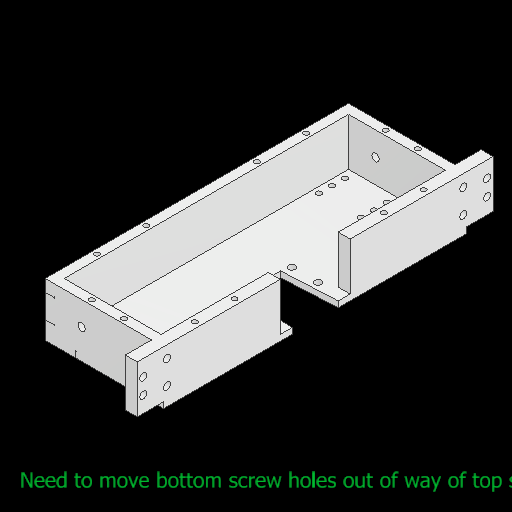
# Autodesk Inventor part: AfterComp1Chassis
Saved by Autodesk Inventor 2024.2 (Build 282272000, 272)
## iProperties
Created: 2021-02-15
Part Number: AfterComp1Chassis
Material: UHMW, White
Document SubType Name: Modeling
Designer: Esketitttttt
Density: 0.94 g/cm^3
Appearance: Smooth - White
Mass: 89.3613 g
Surface Area: 481.722 cm^2
Volume: 95.0653 cm^3
ThreadingScrew: 0.110 in
ThroughScrew: 0.150 in
Author: Esketitttttt
Autodesk Inventor part; units mm, degrees
ref_plane "YZ Plane" through (0, 0, 0) normal (1, 0, 0) x (0, 1, 0)
ref_plane "XZ Plane" through (0, 0, 0) normal (0, 1, 0) x (-1, 0, 0)
sketch "BasePlan" plane through (0, 0, 0) normal (0, 1, 0) x (-1, 0, 0)
  line L0 (0, 0) -> (-51.64, 0)
  line L1 (-51.64, 0) -> (-51.64, -24.585)
  line L2 (-51.64, -24.585) -> (0, -24.585)
  line L3 (0, -24.585) -> (0, 0)
  line L4 (0, 0) -> (-28.78, 0)
  line L5 (-28.78, 0) -> (-28.78, 63.5)
  line L6 (-28.78, 63.5) -> (0, 63.5)
  line L7 (0, 63.5) -> (0, 0)
  line L8 (-28.78, 63.5) -> (-51.64, 63.5)
  line L9 (-51.64, 63.5) -> (-51.64, 0)
  line L10 (-51.64, 0) -> (-28.78, 0)
  line L11 (-28.78, 0) -> (-28.78, 63.5)
  line L12 (0, 0) -> (0, -12.2925)
  line L13 (0, -12.2925) -> (8.9825, -12.2925) construction
  line L14 (-28.78, -24.585) -> (-28.78, -88.085)
  line L15 (-28.78, -88.085) -> (0, -88.085)
  line L16 (0, -88.085) -> (0, -24.585)
  line L17 (-28.78, -88.085) -> (-51.64, -88.085)
  line L18 (-51.64, -88.085) -> (-51.64, -24.585)
  line L19 (0, -88.085) -> (6.35, -88.085) construction
  line L20 (6.35, -88.085) -> (6.35, -94.435) construction
  line L21 (6.35, -94.435) -> (0, -94.435) construction
  line L22 (0, -94.435) -> (0, -88.085) construction
  line L23 (0, 63.5) -> (6.35, 63.5) construction
  line L24 (6.35, 63.5) -> (6.35, 69.85) construction
  line L25 (6.35, 69.85) -> (0, 69.85) construction
  line L26 (0, 69.85) -> (0, 63.5) construction
  line L27 (-51.64, -88.085) -> (-57.99, -88.085) construction
  line L28 (-57.99, -88.085) -> (-57.99, -94.435) construction
  line L29 (-57.99, -94.435) -> (-51.64, -94.435) construction
  line L30 (-51.64, -94.435) -> (-51.64, -88.085) construction
  line L31 (-51.64, 63.5) -> (-57.99, 63.5) construction
  line L32 (-57.99, 63.5) -> (-57.99, 69.85) construction
  line L33 (-57.99, 69.85) -> (-51.64, 69.85) construction
  line L34 (-51.64, 69.85) -> (-51.64, 63.5) construction
  line L35 (-57.99, 69.85) -> (-51.64, 69.85)
  line L36 (-51.64, 69.85) -> (-51.64, 0)
  line L37 (-51.64, 0) -> (-57.99, 0)
  line L38 (-57.99, 0) -> (-57.99, 69.85)
  line L39 (6.35, 69.85) -> (0, 69.85)
  line L40 (0, 69.85) -> (0, -94.435)
  line L41 (0, -94.435) -> (6.35, -94.435)
  line L42 (6.35, -94.435) -> (6.35, 69.85)
  line L43 (-51.64, 69.85) -> (0, 69.85)
  line L44 (0, 69.85) -> (0, 63.5)
  line L45 (0, 63.5) -> (-51.64, 63.5)
  line L46 (-51.64, 63.5) -> (-51.64, 69.85)
  line L47 (-51.64, -88.085) -> (0, -88.085)
  line L48 (0, -88.085) -> (0, -94.435)
  line L49 (0, -94.435) -> (-51.64, -94.435)
  line L50 (-51.64, -94.435) -> (-51.64, -88.085)
  line L51 (-57.99, -94.435) -> (-51.64, -94.435)
  line L52 (-51.64, -94.435) -> (-51.64, -24.585)
  line L53 (-51.64, -24.585) -> (-57.99, -24.585)
  line L54 (-57.99, -24.585) -> (-57.99, -94.435)
  line L55 (-51.64, -24.585) -> (-57.99, -24.585)
  line L56 (-57.99, -24.585) -> (-57.99, -30.935)
  line L57 (-57.99, -30.935) -> (-51.64, -30.935)
  line L58 (-51.64, -30.935) -> (-51.64, -24.585)
  line L59 (-51.64, 0) -> (-57.99, 0)
  line L60 (-57.99, 0) -> (-57.99, 6.35)
  line L61 (-57.99, 6.35) -> (-51.64, 6.35)
  line L62 (-51.64, 6.35) -> (-51.64, 0)
  line L63 (-51.64, 69.85) -> (-57.99, 69.85)
  line L64 (-57.99, 69.85) -> (-57.99, 82.55)
  line L65 (-57.99, 82.55) -> (-51.64, 82.55)
  line L66 (-51.64, 82.55) -> (-51.64, 69.85)
  line L67 (-57.99, -94.435) -> (-51.64, -94.435)
  line L68 (-57.99, -94.435) -> (-57.99, -107.135)
  line L69 (-57.99, -107.135) -> (-51.64, -107.135)
  line L70 (-51.64, -107.135) -> (-51.64, -94.435)
  line L71 (-51.64, -12.2925) -> (-28.78, -12.2925) construction
  line L72 (-28.78, -12.2925) -> (-28.78, -23.0875)
  line L73 (-28.78, -12.2925) -> (-28.78, -1.4975)
  line L74 (-57.99, 0) -> (-28.78, -1.4975)
  line L75 (-57.99, -24.585) -> (-28.78, -23.0875)
  line L76 (0, -94.435) -> (5.08, -94.435)
  line L77 (5.08, -94.435) -> (5.08, 69.85)
  line L78 (5.08, 69.85) -> (0, 69.85)
  line L79 (0, 69.85) -> (0, -94.435)
  line L80 (6.35, -88.085) -> (-51.64, -88.085)
  line L81 (-51.64, -88.085) -> (-51.64, -93.165)
  line L82 (-51.64, -93.165) -> (6.35, -93.165)
  line L83 (6.35, -93.165) -> (6.35, -88.085)
  line L84 (6.35, 63.5) -> (-51.64, 63.5)
  line L85 (-51.64, 63.5) -> (-51.64, 68.58)
  line L86 (-51.64, 68.58) -> (6.35, 68.58)
  line L87 (6.35, 68.58) -> (6.35, 63.5)
  line L88 (-57.99, -94.435) -> (-51.64, -94.435)
  line L89 (-51.64, -94.435) -> (-51.64, -93.165)
  line L90 (-51.64, -93.165) -> (-57.99, -93.165)
  line L91 (-57.99, -93.165) -> (-57.99, -94.435)
  line L92 (-51.64, 68.58) -> (-57.99, 68.58)
  line L93 (-57.99, 68.58) -> (-57.99, 69.85)
  line L94 (-57.99, 69.85) -> (-51.64, 69.85)
  line L95 (-51.64, 69.85) -> (-51.64, 68.58)
  point P0 (0, -88.085)
  point P1 (-51.64, 6.35)
  point P2 (-51.64, -30.935)
  point P3 (5.08, -93.165)
  point P4 (5.08, 68.58)
  dimension "d3" = 28.78
  dimension "d5" = 22.86
  dimension "d6" = 24.585
  dimension "d7" = 63.5
  dimension "d8" = 51.64
  dimension "d9" = 51.64
  dimension "d10" = 12.2925
  dimension "d12" = 6.35
  dimension "d88" = 6.35
  dimension "d89" = 6.35
  dimension "d90" = 6.35
  dimension "d158" = 164.285
  dimension "d210" = 12.7
  dimension "d219" = 22.86
  dimension "d220" = 10.795
  dimension "d255" = 6.35
  dimension "d256" = 5.08
  dimension "d261" = 5.08
  dimension "d262" = 5.08
  constraints: 192 end point, 40 parallel, 22 horizontal, 20 perpendicular, 10 symmetric about line, 8 point on line, 6 equal length, 2 midpoint, 2 vertical
  measures "d3" distance of L5.end L6.end
  measures "d5" distance of L5.end L8.end
  measures "d6" distance of L2.end L0.start
  measures "d7" distance of L6.end L0.start
  measures "d8" distance of L8.end L6.end
  measures "d9" distance of L1.end L2.end
  measures "d10" distance of L0.start L12.end
  measures "d12" distance of L19.end L20.end
  measures "d88" distance of L57.end L56.end
  measures "d89" distance of L56.end L55.end
  measures "d90" distance of L59.end L60.end
  measures "d158" distance of L41.end L24.end
  measures "d210" distance of L63.end L64.end
  measures "d219" distance of L71.start L71.end
  measures "d220" distance of L71.end L72.end
  measures "d255" distance between parallel lines of L40 L42
  measures "d256" distance of L78.end L77.end
  measures "d261" distance of L81.end L80.end
  measures "d262" distance of L84.end L85.end
extrude "BackWall" add sketch "BasePlan" along normal blind 25.4 contours L7 L84 L77 L80 L16 L3 | L40 L86 L77 L84 | L40 L39 L77 L86 | L84 L42 L80 L77 | L77 L86 L42 L84 | L80 L77 L82 L40 | L77 L39 L42 L86 | L80 L42 L82 L77 | L82 L77 L41 L40 | L82 L42 L41 L77
sketch "Sketch2" plane through (-6.35, 0, -94.435) normal (-1, 0, 0) x (0, 0, 1)
  line L0 (0, 0) -> (0, 25.4) construction
  line L1 (0, 0) -> (164.285, 0) construction
  line L2 (0, 0) -> (3.175, 0) construction
  line L3 (3.175, 0) -> (3.175, 6.35) construction
  line L4 (3.175, 6.35) -> (0, 6.35) construction
  line L5 (0, 6.35) -> (0, 0) construction
  line L6 (3.175, 0) -> (3.175, 19.05) construction
  line L7 (0, 25.4) -> (164.285, 25.4) projected
  line L8 (0, 25.4) -> (82.1425, 25.4) construction
  line L9 (82.1425, 25.4) -> (82.1425, 53.975) construction
  point P0 (94.435, 0)
  point P1 (6.35, 0)
  point P2 (161.11, 19.05)
  point P3 (161.11, 6.35)
  dimension "d25" = 6.35
  dimension "d26" = 25.4
  dimension "d27" = 3.175
  dimension "d28" = 6.35
  dimension "d29" = 19.05
  dimension "d30" = 164.285
  dimension "d31" = 82.1425
  constraints: 14 end point, 2 coincident, 2 parallel, 2 symmetric about line, 1 horizontal, 1 midpoint, 1 perpendicular, 1 point on line, 1 vertical
  measures "d25" distance of L0.start point (6.35, 0)
  measures "d26" distance of L0.start L0.end
  measures "d27" distance of L4.end L3.end
  measures "d28" distance of L3.end L2.end
  measures "d29" distance of L2.end L6.end
  measures "d30" distance of L0.end L7.end
  measures "d31" distance of L0.end L8.end
extrude "LeftSideWall" add sketch "BasePlan" along normal up to surface (25.4 mm away) contours L40 L82 L50 L17 L15 | L40 L49 L50 L82
extrude "RightSideWall" add sketch "BasePlan" along normal up to surface (25.4 mm away) contours L6 L8 L36 L86 L40 | L86 L36 L43 L40
hole "BackHoles" at (-6.35, 6.35, -91.26) at (-6.35, 19.05, -91.26) at (-6.35, 19.05, 66.675) at (-6.35, 6.35, 66.675) direction (1, 0, 0) diameter 3.81 depth 6.35
hole "Back Threading Holes" at (-6.35, 6.35, -91.26) at (-6.35, 19.05, -91.26) at (-6.35, 19.05, 66.675) at (-6.35, 6.35, 66.675) direction (1, 0, 0) diameter 2.794 depth 12.7 tip angle 118
extrude "RightFrontWall" add sketch "BasePlan" along normal up to surface (25.4 mm away) contours L61 L38 L92 L36 L9 | L92 L38 L35 L36 | L35 L64 L65 L66
extrude "LeftFrontWall" add sketch "BasePlan" along normal up to surface (25.4 mm away) contours L18 L50 L90 L54 L57 | L50 L51 L54 L90 | L70 L69 L68 L51
extrude "BottomUHMW" add sketch "BasePlan" against normal blind 3.175 contours L3 L2 L1 L75 L72 L73 L74 L0 | L7 L84 L77 L80 L16 L3 | L0 L5 L6 L7 | L0 L9 L8 L5 | L6 L8 L36 L86 L40 | L40 L86 L77 L84 | L37 L38 L61 L9 | L1 L74 L37 | L16 L15 L14 L2 | L86 L36 L43 L40 | L40 L39 L77 L86 | L84 L42 L80 L77 | L77 L86 L42 L84 | L61 L38 L92 L36 L9 | L14 L17 L18 L2 | L40 L82 L50 L17 L15 | L80 L77 L82 L40 | L92 L38 L35 L36 | L77 L39 L42 L86 | L80 L42 L82 L77 | L1 L53 L75 | L18 L57 L54 L53 | L82 L77 L41 L40 | L40 L49 L50 L82 | L82 L42 L41 L77 | L18 L50 L90 L54 L57 | L50 L51 L54 L90
sketch "Sketch4" plane through (0, 25.4, 0) normal (0, -1, 0) x (1, 0, 0)
  line L0 (-4.7625, -65.2173) -> (-4.7625, -63.6933) construction
  line L1 (-4.7625, -65.2173) -> (-4.7625, -63.6933) construction
  line L2 (0, -94.435) -> (0, -88.085) construction
  line L3 (-6.35, -96.4725) -> (-6.35, -94.435) construction
  line L4 (-6.35, -91.71) -> (-6.35, -96.4725) construction
  line L5 (0, 63.5) -> (0, -88.085)
  line L6 (0, -12.2925) -> (-7.0758, -12.2925)
  line L7 (54.815, -30.935) -> (57.99, -30.935) construction
  line L8 (57.99, -30.935) -> (57.99, -52.1017) construction
  line L9 (57.99, -52.1017) -> (54.815, -52.1017) construction
  line L10 (54.815, -52.1017) -> (54.815, -30.935) construction
  line L11 (54.815, -78.0308) -> (54.815, -73.2683) construction
  line L12 (-6.35, -94.435) -> (57.99, -94.435)
  line L13 (-6.35, -94.435) -> (57.99, -94.435) projected
  line L14 (-6.35, -94.435) -> (-3.1992, -94.435)
  line L15 (-2.54, -94.435) -> (-2.54, -68.1125) construction
  line L16 (51.64, -88.085) -> (0, -88.085) projected
  line L17 (-2.54, -94.435) -> (-2.54, -41.79) construction
  line L18 (57.99, -94.435) -> (57.99, -24.585) projected
  line L19 (57.99, -30.935) -> (51.64, -30.935) projected
  line L20 (-6.35, -94.435) -> (-6.35, 69.85) projected
  line L21 (-6.35, -94.435) -> (0, -94.435)
  point P0 (-2.54, 43.5275)
  point P1 (50.37, -94.435)
  point P2 (-2.54, 17.205)
  point P3 (57.99, 27.5167)
  point P4 (54.815, 48.6833)
  point P5 (57.99, -30.9122)
  point P6 (54.815, 27.5167)
  dimension "d104" = 4.7625
  dimension "d119" = 26.3225
  dimension "d121" = 82.1425
  dimension "d132" = 52.645
  dimension "d160" = 63.5
  dimension "d161" = 21.1667
  dimension "d162" = 21.1667
  dimension "d195" = 0
  dimension "d257" = 2.54
  dimension "d258" = 164.285
  constraints: 34 end point, 6 coincident, 5 point on line, 5 symmetric about line, 3 midpoint, 3 vertical, 2 parallel, 2 perpendicular, 1 collinear, 1 horizontal, 1 other
  measures "d104" distance of L11.start L11.end
  measures "d119" distance of L15.start L15.end
  measures "d121" distance between parallel lines of L12 L6
  measures "d132" distance of L15.start L17.end
  measures "d160" vertical distance of L7.end point (50.37, -94.435)
  measures "d161" vertical distance of point (54.815, -73.268) point (50.37, -94.435)
  measures "d162" distance of L7.end point (57.99, -52.102)
  measures "d195" distance between parallel lines of L10 L11
  measures "d257" distance between parallel lines of L5 L17
  measures "d258" distance of L3.end L20.end
hole "NewTopHoles" at (-2.54, 25.4, 43.5275) at (-2.54, 25.4, -68.1125) at (54.815, 25.4, -73.2683) at (-2.54, 25.4, -41.79) at (-2.54, 25.4, 17.205) at (54.815, 25.4, 48.6833) at (54.815, 25.4, -52.1017) at (54.815, 25.4, 27.5167) direction (0, -1, 0) diameter 2.794 depth 12.7 tip angle 118
sketch "Sketch5" plane through (0, 25.4, 0) normal (0, 1, 0) x (1, 0, 0)
  line L0 (-6.35, -69.85) -> (-1.5875, -69.85) construction
  line L1 (-1.5875, -69.85) -> (-1.5875, -65.0875) construction
  line L2 (-1.5875, -65.0875) -> (-6.35, -65.0875) construction
  line L3 (-6.35, -65.0875) -> (-6.35, -69.85) construction
  line L4 (-6.35, -65.0875) -> (-3.9687, -65.0875) construction
  line L5 (-3.9687, -65.0875) -> (-3.9687, -60.325) construction
  line L6 (-3.9687, -60.325) -> (-6.35, -60.325) construction
  line L7 (-6.35, -60.325) -> (-6.35, -65.0875) construction
  line L8 (24.5823, -62.6052) -> (26.9114, -66.7594)
  line L9 (20.7687, 12.2925) -> (-4.7625, 12.2925)
  line L10 (-6.35, -69.85) -> (51.64, -69.85) projected
  line L11 (-6.35, 94.435) -> (-6.35, -69.85) projected
  line L12 (-6.35, 12.2925) -> (-15.875, 12.2925)
  line L13 (37.5312, -37.0575) -> (37.5312, -32.295) construction
  line L14 (-86.3753, 38.7077) -> (-86.3753, 33.9452) construction
  circle A0 centre (54.815, 71.1289) radius 1.4732 projected
  circle A1 centre (38.8013, -32.295) radius 1.0922 projected
  point P0 (0, 0)
  point P1 (-3.9687, 84.91)
  point P2 (-3.9687, 84.91)
  point P3 (57.99, -63.5)
  dimension "d63" = 17.7775
  dimension "d64" = 2.3813
  dimension "d65" = 4.7625
  dimension "d66" = 0
  dimension "d106" = 4.7625
  dimension "d107" = 4.7625
  constraints: 26 end point, 6 symmetric about line, 4 coincident, 4 parallel, 3 horizontal, 2 perpendicular, 2 vertical, 3 other
  measures "d64" distance of L6.end L5.end
  measures "d65" distance of L5.end L4.end
  measures "d66" distance between parallel lines of L12 L9
  measures "d106" distance of L13.start L13.end
  measures "d107" distance of L14.start L14.end
hole "TopHoles" [suppressed]
sketch "Sketch6" plane through (57.99, 1.5875, 103.2682) normal (1, 0, 0) x (0, 0, -1)
  line L0 (33.4182, -1.5875) -> (33.4182, 23.8125) construction
  line L1 (0, 0) -> (146.8373, -1.5875) construction
  line L2 (33.4182, -1.5875) -> (36.5932, -1.5875) construction
  line L3 (36.5932, -1.5875) -> (36.5932, 4.7625) construction
  line L4 (36.5932, 4.7625) -> (33.4182, 4.7625) construction
  line L5 (33.4182, 4.7625) -> (33.4182, -1.5875) construction
  line L6 (36.5932, -1.5875) -> (36.5932, 17.4625) construction
  line L7 (33.4182, 23.8125) -> (197.7033, 23.8125)
  line L8 (0, 25.4) -> (57.8525, 25.4) construction
  line L9 (57.8525, 25.4) -> (57.8525, 53.975) construction
  line L10 (115.5608, 23.8125) -> (115.5608, 30.162)
  line L11 (191.3304, -1.5875) -> (191.3304, -4.7625) projected
  line L12 (33.4182, -1.5875) -> (33.4182, -4.7625) projected
  point P0 (66.8365, 0)
  point P1 (27.0699, -1.4434)
  point P2 (146.8372, -1.5875)
  point P3 (0, 0)
  point P4 (194.5283, 17.4625)
  point P5 (194.5283, 4.7625)
  point P6 (197.7033, -4.7625)
  point P7 (197.7033, -1.5875)
  dimension "d85" = 6.35
  dimension "d86" = 25.4
  dimension "d77" = 3.175
  dimension "d78" = 6.35
  dimension "d76" = 19.05
  dimension "d75" = 57.8525
  dimension "d164" = 157.9122
  constraints: 20 end point, 3 vertical, 2 coincident, 2 parallel, 2 symmetric about line, 1 horizontal, 1 midpoint, 1 perpendicular, 1 point on line, 4 other
  measures "d85" distance of L0.start point (27.07, -1.443)
  measures "d86" distance of L0.end L0.start
  measures "d77" distance of L4.end L3.end
  measures "d78" distance of L3.end L2.end
  measures "d76" distance of L2.end L6.end
  measures "d75" distance of L8.start L8.end
hole "Front Holes" at (57.99, 6.35, 66.675) at (57.99, 19.05, 66.675) at (57.99, 19.05, -91.26) at (57.99, 6.35, -91.26) direction (-1, 0, 0) diameter 3.81 depth 6.35
hole "Front Threading Holes" at (57.99, 19.05, 66.675) at (57.99, 6.35, 66.675) at (57.99, 6.35, -91.26) at (57.99, 19.05, -91.26) direction (-1, 0, 0) diameter 2.794 depth 12.7 tip angle 118
sketch "Sketch7" plane through (51.64, 25.4, 63.5) normal (0, 0, -1) x (-1, 0, 0)
  line L0 (37.25, -22.225) -> (37.25, -12.7) construction
  line L1 (37.25, -12.7) -> (51.64, -12.7) construction
  line L2 (51.64, -12.7) -> (51.64, -25.4)
  circle A0 centre (37.25, -12.7) radius 8.04 construction
  circle A1 centre (37.25, -12.7) radius 2.96
  line L3 (37.25, -12.7) -> (37.25, -7.2) construction
  line L4 (37.25, -12.7) -> (37.25, -18.2) construction
  circle A2 centre (37.25, -18.2) radius 1.143
  circle A3 centre (37.25, -7.2) radius 1.143
  circle A4 centre (37.25, -12.7) radius 2
  line L5 (35.15, -9.525) -> (27.11, -9.525) construction
  line L6 (51.64, 0) -> (51.64, -25.4) projected
  dimension "d93" = 14.39
  dimension "d94" = 5.5
  dimension "d95" = 5.5
  dimension "d96" = 2.286
  dimension "d97" = 2.286
  dimension "d98" = 4
  dimension "d101" = 12.7
  dimension "d194" = 0
  constraints: 12 end point, 5 centre point, 5 coincident, 1 horizontal, 1 parallel, 1 vertical
  measures "d93" distance of L3.start L1.end
  measures "d94" distance of L3.start L3.end
  measures "d95" distance of L3.start L4.end
  measures "d96" diameter of A2
  measures "d97" diameter of A3
  measures "d98" diameter of A4
  measures "d101" distance of L1.end L2.end
  measures "d194" distance between parallel lines of L2 L6
extrude "MotorHole" cut sketch "Sketch7" along normal through all both and the other way through all contours A4
sketch "Sketch8" plane through (0, -3.175, 0) normal (0, -1, 0) x (1, 0, 0)
  line L0 (16.238, -24.585) -> (16.238, -30.935)
  line L1 (16.238, -27.76) -> (30.1553, -27.76) construction
  line L2 (30.1553, -27.76) -> (44.0727, -27.76) construction
  line L3 (57.99, -24.585) -> (57.99, 0)
  line L4 (57.99, -12.2925) -> (39.7101, -12.2925)
  line L5 (16.238, 3.175) -> (30.1553, 3.175) construction
  line L6 (30.1553, 3.175) -> (44.0727, 3.175) construction
  line L7 (57.99, -30.935) -> (51.64, -30.935) projected
  line L8 (16.238, -30.935) -> (57.99, -30.935)
  line L9 (57.99, -94.435) -> (57.99, -24.585) projected
  point P0 (0, 0)
  point P1 (0, 44.9224)
  point P2 (51.64, -37.2622)
  dimension "d109" = 13.9173
  dimension "d110" = 13.9173
  dimension "d196" = 3.175
  dimension "d197" = 3.175
  dimension "d198" = 3.175
  dimension "d200" = 13.9173
  constraints: 16 end point, 5 coincident, 5 symmetric about line, 2 horizontal, 2 midpoint, 2 vertical, 1 other
  measures "d109" distance of L1.start L1.end
  measures "d110" distance of L1.end L2.end
  measures "d196" distance from line of L8 L2.end
  measures "d197" distance from line of point (30.155, -27.76) L8
  measures "d198" distance of L0.end L1.start
  measures "d200" distance from line of L9 L2.end
hole "UprightHoles" at (30.1553, -3.175, -27.76) at (44.0727, -3.175, -27.76) at (44.0727, -3.175, 3.175) at (30.1553, -3.175, 3.175) direction (0, 1, 0) diameter 3.81 depth 9.525 tip angle 118
sketch "Sketch9" plane through (0, 25.4, 0) normal (0, -1, 0) x (1, 0, 0)
  line L0 (0, 63.5) -> (51.64, 63.5) construction
  line L1 (51.64, -88.085) -> (0, -88.085) construction
  line L2 (-6.35, -94.435) -> (51.64, -94.435) construction
  line L3 (-6.35, 69.85) -> (51.64, 69.85) construction
  line L4 (51.64, 57.15) -> (51.64, 6.35) construction
  line L5 (0, 63.5) -> (0, -88.085) construction
  line L6 (0, -88.085) -> (51.64, -88.085) construction
  line L7 (-6.35, -94.435) -> (57.99, -94.435) construction
  line L8 (0, -88.085) -> (0, -94.435) construction
  line L9 (0, 63.5) -> (0, 63.5) construction
  line L10 (51.64, 57.15) -> (51.64, 69.85) construction
  line L11 (51.64, -90.625) -> (34.4267, -90.625) construction
  line L12 (34.4267, -90.625) -> (17.2133, -90.625) construction
  line L13 (0, -12.2925) -> (7.9375, -12.2925)
  line L14 (-6.35, 69.85) -> (-6.35, -94.435) projected
  point P0 (0, 0)
  point P1 (17.2133, 66.04)
  point P2 (34.4267, 66.04)
  dimension "d123" = 17.2133
  dimension "d124" = 17.2133
  dimension "d163" = 6.35
  dimension "d222" = 51.64
  dimension "d263" = 2.54
  constraints: 14 end point, 3 point on line, 2 coincident, 2 horizontal, 2 perpendicular, 2 symmetric about line, 1 midpoint, 1 parallel, 1 vertical alignment, 1 other
  measures "d123" distance of L11.start L11.end
  measures "d124" distance of L11.end L12.end
  measures "d163" distance from line of L14 L1.end
  measures "d222" distance of L1.start L1.end
  measures "d263" distance from line of L1 L12.end
hole "SideWallTopHoles" at (17.2133, 25.4, -90.625) at (34.4267, 25.4, -90.625) at (17.2133, 25.4, 66.04) at (34.4267, 25.4, 66.04) direction (0, -1, 0) diameter 2.794 depth 9.525 tip angle 118
ref_plane "MidHeightPlane" through (0, 11.1125, 0) normal (0, 1, 0) x (1, 0, 0)
sketch "Sketch10" plane through (57.99, 25.4, 69.85) normal (1, 0, 0) x (0, 0, -1)
  circle A0 centre (9.525, -16.9333) radius 1.0922
  circle A1 centre (9.525, -8.4667) radius 1.0922
  circle A2 centre (60.325, -8.4667) radius 1.0922
  circle A3 centre (60.325, -16.9333) radius 1.0922
  circle A4 centre (103.96, -16.9333) radius 1.0922
  circle A5 centre (103.96, -8.4667) radius 1.0922
  circle A6 centre (148.3872, -8.4667) radius 1.0922
  circle A7 centre (148.3872, -16.9333) radius 1.0922
  line L0 (41.82, 0) -> (0, 0)
  line L1 (57.15, 0) -> (-12.7, 0) projected
  line L2 (0, -25.4) -> (0, -28.575) projected
  line L3 (63.5, -25.4) -> (63.5, 0) projected
  line L4 (100.785, -25.4) -> (100.785, 0) projected
  line L5 (157.9122, -25.4) -> (157.9122, -28.575) projected
  circle A8 centre (-9.525, -8.4667) radius 1.0922
  circle A9 centre (-9.525, -16.9333) radius 1.0922
  circle A10 centre (173.81, -8.4667) radius 1.0922
  circle A11 centre (173.81, -16.9333) radius 1.0922
  line L6 (-12.7, -25.4) -> (-12.7, 0) projected
  point P0 (57.15, -25.4)
  point P1 (100.7622, -25.4)
  point P2 (164.285, -28.575)
  point P3 (157.9122, 0)
  point P4 (164.285, -25.4)
  point P5 (100.785, 0)
  point P6 (63.5, 0)
  point P7 (176.985, 0)
  dimension "d167" = 9.525
  dimension "d168" = 9.525
  dimension "d169" = 3.175
  dimension "d170" = 3.175
  dimension "d171" = 8.4667
  dimension "d172" = 8.4667
  dimension "d173" = 3.175
  dimension "d174" = 3.175
  dimension "d175" = 9.525
  dimension "d176" = 9.525
  dimension "d177" = 8.4667
  dimension "d178" = 8.4667
  dimension "d180" = 2.1844
  dimension "d181" = 2.1844
  dimension "d182" = 2.1844
  dimension "d183" = 2.1844
  dimension "d184" = 2.1844
  dimension "d185" = 2.1844
  dimension "d186" = 2.1844
  dimension "d187" = 2.1844
  dimension "d208" = 25.4
  dimension "d209" = 28.575
  dimension "d211" = 2.1844
  dimension "d212" = 2.1844
  dimension "d213" = 2.1844
  dimension "d214" = 2.1844
  dimension "d215" = 8.4667
  dimension "d216" = 8.4667
  dimension "d217" = 3.175
  dimension "d254" = 3.175
  constraints: 12 centre point, 5 horizontal alignment, 4 coincident, 2 end point, 2 vertical alignment, 3 other
  measures "d167" distance from line of L2 A1.centre
  measures "d168" distance from line of L2 A0.centre
  measures "d171" distance of A3.centre A2.centre
  measures "d172" distance of A0.centre A1.centre
  measures "d177" distance of A7.centre A6.centre
  measures "d178" distance from line of L1 A1.centre
  measures "d180" diameter of A7
  measures "d181" diameter of A6
  measures "d182" diameter of A5
  measures "d183" diameter of A4
  measures "d184" diameter of A3
  measures "d185" diameter of A2
  measures "d186" diameter of A0
  measures "d187" diameter of A1
  measures "d208" distance of point (57.15, -25.4) L1.start
  measures "d209" distance of point (0, 0) L2.end
  measures "d211" diameter of A8
  measures "d212" diameter of A9
  measures "d213" diameter of A10
  measures "d214" diameter of A11
  measures "d215" distance from line of L1 A8.centre
  measures "d216" distance of A9.centre A8.centre
  measures "d217" distance from line of L6 A8.centre
  measures "d254" horizontal distance of point (176.985, 0) point (173.81, -8.467)
hole "WedgeletHoles" at (57.99, 16.9333, -103.96) at (57.99, 8.4667, -103.96) at (57.99, 8.4667, 79.375) at (57.99, 16.9333, 79.375) direction (-1, 0, 0) diameter 3.81 depth 6.35 tip angle 118
sketch "Sketch11" plane through (0, -3.175, 0) normal (0, -1, 0) x (1, 0, 0)
  line L0 (-6.35, -94.435) -> (-6.35, 69.85) projected
  line L1 (-6.35, 69.85) -> (57.99, 69.85)
  line L2 (57.99, 69.85) -> (57.99, -94.435)
  line L3 (51.64, -88.085) -> (51.64, 63.5)
  line L4 (51.64, 63.5) -> (0, 63.5)
  line L5 (0, 63.5) -> (0, -88.085)
  line L6 (0, -88.085) -> (51.64, -88.085)
  line L7 (28.78, 39.5) -> (0, 39.5) construction
  line L8 (0, 39.5) -> (0, 63.5)
  line L9 (28.78, 39.5) -> (28.78, 51.5)
  line L10 (0, 51.5) -> (0, 39.5)
  line L11 (28.78, 39.5) -> (28.78, 63.5)
  line L12 (28.78, 39.345) -> (28.78, 63.5)
  line L13 (28.78, 39.5) -> (28.78, 45.5)
  line L14 (28.78, 63.5) -> (0, 63.5)
  line L15 (51.64, 4.3636) -> (51.64, -28.9486)
  line L16 (51.64, -12.2925) -> (32.0322, -12.2925)
  line L17 (51.64, -12.2925) -> (71.2478, -12.2925) construction
  line L18 (0, 39.5) -> (3.175, 39.5)
  line L19 (28.78, 39.5) -> (25.605, 39.5)
  line L20 (25.605, 39.5) -> (25.605, 51.5) construction
  line L21 (14.39, 39.5) -> (14.39, 42.5) construction
  line L22 (25.605, 51.5) -> (25.605, 44.625) construction
  line L23 (25.605, 51.5) -> (25.605, 58.375) construction
  line L24 (-6.35, -94.435) -> (57.99, -94.435) projected
  line L25 (-6.35, -94.435) -> (57.99, -94.435)
  point P0 (0, 0)
  point P1 (3.175, 58.375)
  point P2 (3.175, 51.5)
  point P3 (3.175, 44.625)
  point P4 (25.605, -82.96)
  point P5 (25.605, -82.96)
  point P6 (25.605, -76.085)
  point P7 (25.605, -69.21)
  point P8 (3.175, -69.21)
  point P9 (3.175, -76.085)
  point P10 (3.175, -82.96)
  dimension "d140" = 6.35
  dimension "d150" = 180
  dimension "d189" = 0
  dimension "d190" = 0
  dimension "d201" = 28.78
  dimension "d202" = 24
  dimension "d203" = 3.175
  dimension "d204" = 3.175
  dimension "d205" = 12
  dimension "d206" = 6.875
  dimension "d207" = 6.875
  dimension "d225" = 6.35
  constraints: 48 end point, 10 symmetric about line, 5 coincident, 5 midpoint, 4 equal length, 4 vertical, 3 perpendicular, 3 point on line, 2 horizontal, 1 collinear, 1 other
  measures "d140" distance between parallel lines of L2 L3
  measures "d150" angle of L16 L17
  measures "d189" distance between parallel lines of L4 L14
  measures "d190" distance between parallel lines of L5 L8
  measures "d201" distance between parallel lines of L13 L5
  measures "d202" distance between parallel lines of L14 L7
  measures "d203" distance of L10.end L18.end
  measures "d204" distance of L11.start L19.end
  measures "d205" distance of L19.end L20.end
  measures "d206" distance of L20.end L22.end
  measures "d207" distance of L20.end L23.end
  measures "d225" distance between parallel lines of L6 L24
hole "BottomMotorMountHoles" at (25.605, -3.175, 58.375) at (25.605, -3.175, 51.5) at (25.605, -3.175, 44.625) at (3.175, -3.175, 58.375) at (3.175, -3.175, 51.5) at (3.175, -3.175, 44.625) at (3.175, -3.175, -69.21) at (3.175, -3.175, -76.085) at (3.175, -3.175, -82.96) at (25.605, -3.175, -82.96) at (25.605, -3.175, -76.085) at (25.605, -3.175, -69.21) direction (0, 1, 0) diameter 3 depth 9.525 tip angle 118
sketch "Sketch16" plane through (0, -3.175, 0) normal (0, -1, 0) x (1, 0, 0)
  circle A0 centre (17.2133, 66.04) radius 1.397 construction
  circle A1 centre (17.2133, -90.625) radius 1.397 construction
  circle A2 centre (34.4267, -90.625) radius 1.397 construction
  circle A3 centre (34.4267, 66.04) radius 1.397 construction
  circle A4 centre (54.815, -52.1017) radius 1.397 construction
  circle A5 centre (-2.54, 17.205) radius 1.397 construction
  circle A6 centre (54.815, -73.2683) radius 1.397 construction
  circle A7 centre (-2.54, 43.5275) radius 1.397 construction
  circle A8 centre (-2.54, -68.1125) radius 1.397 construction
  circle A9 centre (-2.54, -41.79) radius 1.397 construction
  circle A10 centre (54.815, 48.6833) radius 1.397 construction
  circle A11 centre (54.815, 27.5167) radius 1.397 construction
  line L0 (-6.35, -94.435) -> (-6.35, 69.85) construction
  line L1 (-6.35, 69.85) -> (51.64, 69.85) construction
  line L2 (51.64, 82.55) -> (51.64, 69.85) construction
  line L3 (57.99, 82.55) -> (51.64, 82.55) construction
  line L4 (57.99, 6.35) -> (57.99, 82.55) construction
  line L5 (51.64, 6.35) -> (57.99, 6.35) construction
  line L6 (51.64, 63.5) -> (51.64, 6.35) construction
  line L7 (0, 63.5) -> (51.64, 63.5) construction
  line L8 (0, 63.5) -> (0, -88.085) construction
  line L9 (51.64, -88.085) -> (0, -88.085) construction
  line L10 (51.64, -30.935) -> (51.64, -88.085) construction
  line L11 (57.99, -30.935) -> (51.64, -30.935) construction
  line L12 (57.99, -107.135) -> (57.99, -30.935) construction
  line L13 (51.64, -107.135) -> (57.99, -107.135) construction
  line L14 (51.64, -94.435) -> (51.64, -107.135) construction
  line L15 (-6.35, -94.435) -> (51.64, -94.435) construction
  line L16 (0, -93.165) -> (0, -89.355) construction
  line L17 (51.64, -89.355) -> (51.64, -93.165) construction
  line L18 (58.2437, -90.625) -> (54.815, -90.625) construction
  line L19 (-1.5068, -88.72) -> (-2.54, -88.72) construction
  circle A12 centre (34.4267, -90.625) radius 1.397 construction
  circle A13 centre (54.815, -73.2683) radius 1.397 construction
  line L20 (54.815, -73.2683) -> (54.815, -90.625) construction
  line L21 (-2.54, -88.72) -> (-2.54, -68.1125) construction
  line L22 (0, 63.5) -> (0, -88.085) projected
  line L23 (0, -12.2925) -> (6.35, -12.2925)
  circle A14 centre (-2.54, -68.1125) radius 1.397 construction
  circle A15 centre (-2.54, -41.79) radius 1.397 construction
  line L24 (-2.54, -68.1125) -> (-2.54, -41.79) construction
  circle A16 centre (-2.54, 17.205) radius 1.397 construction
  line L25 (-2.54, -41.79) -> (-2.54, 17.205) construction
  line L26 (54.815, -73.2683) -> (54.815, -52.1017) construction
  line L27 (54.815, -52.1017) -> (54.815, -30.935) construction
  line L28 (51.64, -30.935) -> (57.99, -30.935) construction
  circle A17 centre (17.2133, -90.625) radius 1.397 projected
  line L29 (0, -93.165) -> (0, -89.355) projected
  circle A18 centre (34.4267, -90.625) radius 1.397 projected
  circle A19 centre (17.2133, -90.625) radius 1.397 construction
  line L30 (51.64, -89.863) -> (51.64, -92.657) construction
  line L31 (45.29, -92.657) -> (45.29, -89.863) construction
  line L32 (6.35, -89.863) -> (6.35, -92.657) construction
  line L33 (6.35, -89.863) -> (6.35, -92.657) projected
  line L34 (6.35, -91.26) -> (15.969, -91.26) construction
  line L35 (45.29, -91.26) -> (35.671, -91.26) construction
  point P0 (0, 0)
  point P1 (-2.54, -78.4163)
  point P2 (54.815, -81.9467)
  point P3 (40.4805, -91.26)
  point P4 (11.1595, -91.26)
  point P5 (-2.54, 53.8312)
  point P6 (54.815, 57.3617)
  point P7 (40.4805, 66.675)
  point P8 (11.1595, 66.675)
  point P9 (54.815, -62.685)
  point P10 (54.815, -41.5183)
  point P11 (-2.54, -54.9513)
  point P12 (-2.54, -12.2925)
  point P13 (54.815, 38.1)
  point P14 (54.815, 16.9333)
  point P15 (-2.54, 30.3662)
  constraints: 22 end point, 12 midpoint, 7 symmetric about line, 4 horizontal, 3 vertical, 2 perpendicular, 2 vertical alignment, 1 collinear, 1 horizontal alignment, 4 other
hole "BottomHoles" at (-2.54, -3.175, -78.4163) at (54.815, -3.175, -81.9467) at (40.4805, -3.175, -91.26) at (11.1595, -3.175, -91.26) at (-2.54, -3.175, 53.8312) at (11.1595, -3.175, 66.675) at (40.4805, -3.175, 66.675) at (54.815, -3.175, 57.3617) at (54.815, -3.175, -62.685) at (54.815, -3.175, -41.5183) at (-2.54, -3.175, -54.9513) at (-2.54, -3.175, -12.2925) at (-2.54, -3.175, 30.3662) at (54.815, -3.175, 16.9333) at (54.815, -3.175, 38.1) direction (0, 1, 0) diameter 3.81 depth 3.175
hole "BottomThreadingHoles" at (54.815, -3.175, 57.3617) at (54.815, -3.175, 38.1) at (54.815, -3.175, 16.9333) at (54.815, -3.175, -41.5183) at (54.815, -3.175, -62.685) at (54.815, -3.175, -81.9467) at (40.4805, -3.175, 66.675) at (11.1595, -3.175, 66.675) at (-2.54, -3.175, -12.2925) at (-2.54, -3.175, 30.3662) at (-2.54, -3.175, 53.8312) at (-2.54, -3.175, -54.9513) at (-2.54, -3.175, -78.4163) at (11.1595, -3.175, -91.26) at (40.4805, -3.175, -91.26) direction (0, 1, 0) diameter 2.794 depth 12.7 tip angle 118
extrude "JankFix" cut sketch "BasePlan" along normal through all both and the other way through all contours L86 L36 L43 L40 | L40 L39 L77 L86 | L84 L42 L80 L77 | L77 L86 L42 L84 | L77 L39 L42 L86 | L80 L42 L82 L77 | L82 L77 L41 L40 | L40 L49 L50 L82 | L82 L42 L41 L77
extrude "jankj2222" cut sketch "BasePlan" against normal through all contours L92 L38 L35 L36 | L50 L51 L54 L90
equation "\"d9\" = d8"
equation "\"d10\" = 0.5 * d6"
equation "\"d27\" = 0.5 * d25"
equation "\"d28\" = 0.25 * d26"
equation "\"d29\" = 3 * d28"
equation "\"d31\" = 0.5 * d30"
equation "\"d77\" = 0.5 * d85"
equation "\"d78\" = 0.25 * d86"
equation "\"d76\" = 3 * d78"
body "Solid1"
